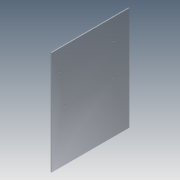
# Autodesk Inventor part: mount
Saved by Autodesk Inventor 2015 SP1 (Build 190203100, 203)
## iProperties
Created: 2015-07-22
Part Number: mount
Material: Generic
Document SubType Name: Modeling
Designer: James
Density: 1 g/cm^3
Appearance: Clear
Author: James
Autodesk Inventor part; units mm, degrees
ref_plane "YZ Plane" through (0, 0, 0) normal (1, 0, 0) x (0, 1, 0)
ref_plane "XZ Plane" through (0, 0, 0) normal (0, 1, 0) x (-1, 0, 0)
ref_plane "XY Plane" through (0, 0, 0) normal (0, 0, 1) x (1, 0, 0)
sketch "Sketch1" plane through (0, 0, 0) normal (1, 0, 0) x (0, 1, 0)
  line L0 (69.1948, 82.7013) -> (-50.8052, 82.7013)
  line L1 (-50.8052, 82.7013) -> (-50.8052, -77.2987)
  line L2 (-50.8052, -77.2987) -> (69.1948, -77.2987)
  line L3 (69.1948, -77.2987) -> (69.1948, 82.7013)
  point P0 (0, 0)
  dimension "d0" = 160
  dimension "d1" = 120
  constraints: 8 end point, 2 parallel, 1 horizontal, 1 perpendicular
  measures "d0" distance between parallel lines of L0 L2
  measures "d1" distance between parallel lines of L3 L1
extrude "Extrusion1" add sketch "Sketch1" along normal blind 1.5
sketch "Sketch2" plane through (1.5, 0, 0) normal (1, 0, 0) x (0, 0, -1)
  line L0 (-52.7013, 59.1948) -> (0.5987, 59.1948)
  line L1 (-52.7013, 59.1948) -> (-52.7013, -42.4052)
  line L2 (77.2987, 69.1948) -> (-82.7013, 69.1948) projected
  line L3 (-82.7013, 69.1948) -> (-82.7013, -50.8052) projected
  line L4 (0.5987, 59.1948) -> (0.5987, -42.4052)
  line L5 (0.5987, -42.4052) -> (-52.7013, -42.4052)
  point P0 (0, 0)
  point P1 (-50.2013, 45.1948)
  point P2 (-50.2013, -37.3252)
  point P3 (-2.0013, 43.8948)
  point P4 (-2.0013, -31.0052)
  dimension "d4" = 14
  dimension "d5" = 15.3
  dimension "d6" = 101.6
  dimension "d7" = 2.5
  dimension "d8" = 10
  dimension "d9" = 30
  dimension "d10" = 53.3
  dimension "d12" = 2.5
  dimension "d13" = 50.7
  dimension "d14" = 50.7
  dimension "d15" = 90.2
  dimension "d16" = 96.52
  constraints: 8 end point, 2 vertical, 1 horizontal, 1 perpendicular
  measures "d4" distance from line of point (-50.201, 45.195) L0
  measures "d5" distance from line of point (-2.001, 43.895) L0
  measures "d6" distance of L0.start L1.end
  measures "d7" distance from line of point (-50.201, 45.195) L1
  measures "d8" distance between parallel lines of L2 L0
  measures "d9" distance between parallel lines of L3 L1
  measures "d10" distance of L0.start L0.end
  measures "d12" distance from line of L1 point (-50.201, -37.325)
  measures "d13" distance from line of point (-2.001, -31.005) L1
  measures "d14" distance from line of L1 point (-2.001, 43.895)
  measures "d15" distance from line of point (-2.001, -31.005) L0
  measures "d16" distance from line of L0 point (-50.201, -37.325)
hole "Hole1" at (1.5, 45.1948, 50.2013) at (1.5, -37.3252, 50.2013) at (1.5, 43.8948, 2.0013) at (1.5, -31.0052, 2.0013) direction (-1, 0, 0) diameter 2.013 end through all thread size "M2.5x0.45" class "6H" standard "ANSI Metric M Profile"
equation "\"d14\" = d13"
body "Solid1"
